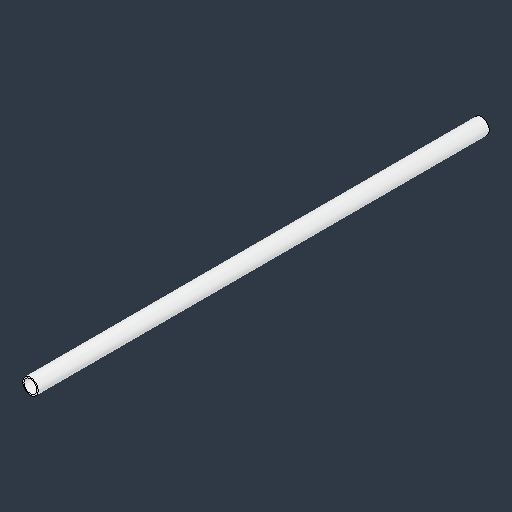
# Autodesk Inventor part: TUBE,ROLLER,LONG
Saved by Autodesk Inventor 2026 (Build 300175050, 175E)
## iProperties
Created: 2026-04-04
Part Number: TUBE,ROLLER,LONG
Material: Aluminum 6061
Document SubType Name: Modeling
Designer: Jthib
Mass: 129.159 g
Surface Area: 604.407 cm^2
Volume: 47.8366 cm^3
Density: 2.7 g/cm^3
Appearance: Aluminum - Flat
Author: Jthib
Autodesk Inventor part; units mm, degrees
ref_plane "YZ Plane" through (0, 0, 0) normal (1, 0, 0) x (0, 1, 0)
ref_plane "XZ Plane" through (0, 0, 0) normal (0, 1, 0) x (-1, 0, 0)
ref_plane "XY Plane" through (0, 0, 0) normal (0, 0, 1) x (1, 0, 0)
sketch "Sketch1" plane through (0, 0, 0) normal (0, 0, 1) x (1, 0, 0)
  circle A0 centre (0, 0) radius 9.525
  circle A1 centre (0, 0) radius 7.9375
  dimension "d0" = 19.05
  dimension "d1" = 15.875
  constraints: 2 centre point, 2 coincident
  measures "d0" diameter of A0
  measures "d1" diameter of A1
extrude "Extrusion1" add sketch "Sketch1" along normal mid plane 549.275
sketch "Sketch2" plane through (0, 0, 274.6375) normal (0, 0, 1) x (1, 0, 0)
  circle A0 centre (0, 0) radius 11.938 construction
  circle A1 centre (0, 0) radius 49.4284 construction
  dimension "d4" = 23.876
  dimension "d6" = 49.4284
  constraints: 2 centre point, 2 coincident
  measures "d4" diameter of A0
  measures "d6" radius of A1
body "Solid1"
